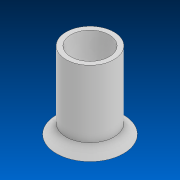
# Autodesk Inventor part: Drill Bit Guide
Saved by Autodesk Inventor 2022.2 (Build 262287000, 287)
## iProperties
Created: 2022-03-25
Part Number: Drill Bit Guide
Material: Generic
Document SubType Name: Modeling
Designer: omard
Density: 1 g/cm^3
Appearance: Default
Author: omard
Autodesk Inventor part; units mm, degrees
ref_plane "YZ Plane" through (0, 0, 0) normal (1, 0, 0) x (0, 1, 0)
ref_plane "XZ Plane" through (0, 0, 0) normal (0, 1, 0) x (-1, 0, 0)
ref_plane "XY Plane" through (0, 0, 0) normal (0, 0, 1) x (1, 0, 0)
sketch "Sketch2" plane through (0, 0, 0) normal (0, 0, 1) x (1, 0, 0)
  line L0 (0, 0) -> (0, 50.8) construction
  line L1 (0, 50.8) -> (12.7, 50.8) construction
  line L2 (12.7, 50.8) -> (12.7, 0)
  line L3 (12.7, 0) -> (0, 0) construction
  line L4 (12.7, 50.8) -> (15.875, 50.8)
  line L5 (15.875, 50.8) -> (15.875, 0)
  line L6 (15.875, 0) -> (12.7, 0)
  line L7 (12.7, 0) -> (12.7, 50.8)
  line L8 (15.875, 0) -> (22.225, 0)
  line L9 (22.225, 0) -> (15.875, 6.35)
  dimension "d3" = 50.8
  dimension "d4" = 12.7
  dimension "d5" = 3.175
  dimension "d6" = 45
  dimension "d7" = 6.35
  constraints: 20 end point, 4 perpendicular, 2 horizontal, 2 parallel, 1 collinear, 1 point on line, 1 vertical
  measures "d3" distance of L0.start L0.end
  measures "d4" distance of L0.end L1.end
  measures "d5" distance of L5.end L6.end
  measures "d6" angle of L8 L9
  measures "d7" distance of L5.end L8.end
revolve "Revolution1" add sketch "Sketch2" angle 360 about axis through (0, 0, 0) along (0, 1, 0)
body "Solid1"
